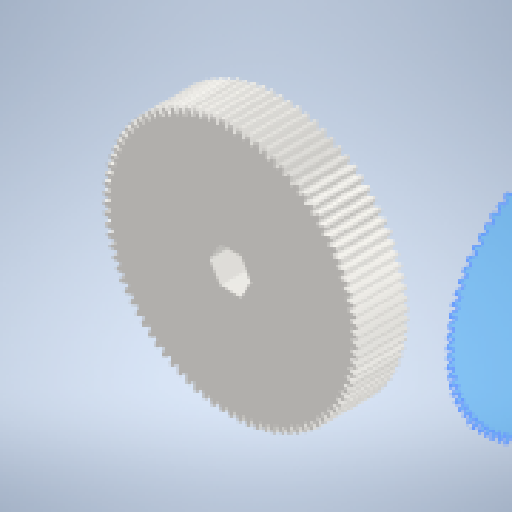
# Autodesk Inventor part: Spur Gear2
Saved by Autodesk Inventor 2024 (Build 280153020, 153B)
## iProperties
CustomPartVersion: 1
Created: 2024-04-17
Part Number: Spur Gear2
Material: Steel
Document SubType Name: Modeling
Designer: lvrectanus0
Categories: <?xml version="1.0" encoding="UTF-16"?> <MemberInstance><Categories><FamilyTemplate><FamilyTemplateParameter ValueType="xs:double" Id="1" ObjectReferenceKey="da_z" ObjectType="kUserParameterObject"/><FamilyTemplateParameter ValueType="xs:double" Id="2" ObjectReferenceKey="da_b" ObjectType="kUserParameterObject"/><FamilyTemplateParameter ValueType="xs:double" Id="3" ObjectReferenceKey="da_beta" ObjectType="kUserParameterObject"/><FamilyTemplateParameter ValueType="xs:double" Id="4" ObjectReferenceKey="da_da" ObjectType="kUserParameterObject"/><FamilyTemplateParameter ValueType="xs:double" Id="5" ObjectReferenceKey="da_aw" ObjectType="kUserParameterObject"/><FamilyTemplateParameter ValueType="xs:string" Id="6" ObjectReferenceKey="EAIAABAAAAC/AAAAAAAAAIAAAAAAAAAA" ObjectType="83910656" SubObjectId="SurfaceGeometry"/></FamilyTemplate><ParamToTemplateMap><ParamToTemplate CategoryParameter="//CategoryParameter[@InternalName='046C89C9-8512-4d59-83FE-43B91F4F132A']" TemplateParameter="1"/><ParamToTemplate CategoryParameter="//CategoryParameter[@InternalName='2552DF32-E462-4b46-AEBF-C6C7768E72AC']" TemplateParameter="2"/><ParamToTemplate CategoryParameter="//CategoryParameter[@InternalName='C9EE641D-15FC-4fae-A226-E94C4372FDD7']" TemplateParameter="3"/><ParamToTemplate><ParamToTemplate CategoryParameter="//CategoryParameter[@InternalName='00B6519A-459B-49c7-AD84-2E56D39A5744']" ConstantValue="0.000000"/></ParamToTemplate><ParamToTemplate><ParamToTemplate CategoryParameter="//CategoryParameter[@InternalName='04B31F0E-C7A6-4894-AA32-9629BEFACF47']" ConstantValue="1.000000"/></ParamToTemplate><ParamToTemplate><ParamToTemplate CategoryParameter="//CategoryParameter[@InternalName='43CBEC2E-7847-49e7-A936-2F7889FCB2D9']" ConstantValue="0.250000"/></ParamToTemplate><ParamToTemplate><ParamToTemplate CategoryParameter="//CategoryParameter[@InternalName='B1EFC894-105D-4ebd-86BF-FA20ED196853']" ConstantValue="0.350000"/></ParamToTemplate><ParamToTemplate><ParamToTemplate CategoryParameter="//CategoryParameter[@InternalName='51175063-3D10-4879-93E8-6246FE8B403D']" ConstantValue="2061532430.657340"/></ParamToTemplate><ParamToTemplate><ParamToTemplate CategoryParameter="//CategoryParameter[@InternalName='A3A52E27-4454-46a9-B0BD-C932399B70AF']" ConstantValue="0.300000"/></ParamToTemplate><ParamToTemplate><ParamToTemplate CategoryParameter="//CategoryParameter[@InternalName='91B76062-C214-41d9-B1B9-14D2AB99603D']" ConstantValue="0.079375"/></ParamToTemplate><ParamToTemplate><ParamToTemplate CategoryParameter="//CategoryParameter[@InternalName='374E806E-8B8A-4dda-A9AA-1039D6500AD2']" ConstantValue="12.598425"/></ParamToTemplate><ParamToTemplate><ParamToTemplate CategoryParameter="//CategoryParameter[@InternalName='2D373A89-B862-43d6-8D0B-0CBF12AB9F6C']" ConstantValue="0.349066"/></ParamToTemplate><ParamToTemplate CategoryParameter="//CategoryParameter[@InternalName='37777632-D6A2-4fac-9D53-DB8ACD95C989']" TemplateParameter="4"/><ParamToTemplate CategoryParameter="//CategoryParameter[@InternalName='FD1017F1-B727-4f7e-9707-0F86F1FF9423']" TemplateParameter="5"/><ParamToTemplate><ParamToTemplate CategoryParameter="//CategoryParameter[@InternalName='9E1B4470-B2D3-4ff1-B813-535BB4CDF51A']" ConstantValue="3523220.976809"/></ParamToTemplate><ParamToTemplate><ParamToTemplate CategoryParameter="//CategoryParameter[@InternalName='F8452263-BFF6-458c-9FB1-07C4B99E95CD']" ConstantValue="11397033.805607"/></ParamToTemplate><ParamToTemplate><ParamToTemplate CategoryParameter="//CategoryParameter[@InternalName='3E3BB259-FD49-497f-8171-6EBC954A3479']" ConstantValue="2.000000"/></ParamToTemplate><ParamToTemplate CategoryParameter="//CategoryParameter[@InternalName='27C3BAF2-7550-4e4b-AE2C-0DB134B7D9B7']" TemplateParameter="6"/></ParamToTemplateMap><Category DisplayName="Gear" InternalName="DC85795E-93AB-48d5-8EEE-5A27447B64BD" Mnemonic="Gear"><CategoryParameter DisplayName="z" InternalName="046C89C9-8512-4d59-83FE-43B91F4F132A" Mnemonic="z"/><CategoryParameter DisplayName="b" InternalName="2552DF32-E462-4b46-AEBF-C6C7768E72AC" Mnemonic="b"/><CategoryParameter DisplayName="||b|" InternalName="C9EE641D-15FC-4fae-A226-E94C4372FDD7" Mnemonic="beta"/><CategoryParameter DisplayName="x" InternalName="00B6519A-459B-49c7-AD84-2E56D39A5744" Mnemonic="x"/><CategoryParameter DisplayName="a*" InternalName="04B31F0E-C7A6-4894-AA32-9629BEFACF47" Mnemonic="a"/><CategoryParameter DisplayName="c*" InternalName="43CBEC2E-7847-49e7-A936-2F7889FCB2D9" Mnemonic="c"/><CategoryParameter DisplayName="r|.f|*" InternalName="B1EFC894-105D-4ebd-86BF-FA20ED196853" Mnemonic="rf"/><CategoryParameter DisplayName="E" InternalName="51175063-3D10-4879-93E8-6246FE8B403D" Mnemonic="E"/><CategoryParameter DisplayName="||m|" InternalName="A3A52E27-4454-46a9-B0BD-C932399B70AF" Mnemonic="mi"/><Category DisplayName="SpurGear" InternalName="26C5A22E-A91E-4dfd-A3B3-23CCAFAE1764" Mnemonic="SpurGear"><CategoryParameter DisplayName="m" InternalName="91B76062-C214-41d9-B1B9-14D2AB99603D" Mnemonic="m"/><CategoryParameter DisplayName="P" InternalName="374E806E-8B8A-4dda-A9AA-1039D6500AD2" Mnemonic="PP"/><CategoryParameter DisplayName="||a|" InternalName="2D373A89-B862-43d6-8D0B-0CBF12AB9F6C" Mnemonic="alpha"/><CategoryParameter DisplayName="d|.a|" InternalName="37777632-D6A2-4fac-9D53-DB8ACD95C989" Mnemonic="da"/><CategoryParameter DisplayName="a|.w|" InternalName="FD1017F1-B727-4f7e-9707-0F86F1FF9423" Mnemonic="aw"/><CategoryParameter DisplayName="||s||.Flim|" InternalName="9E1B4470-B2D3-4ff1-B813-535BB4CDF51A" Mnemonic="sFlim"/><CategoryParameter DisplayName="||s||.Hlim|" InternalName="F8452263-BFF6-458c-9FB1-07C4B99E95CD" Mnemonic="sHlim"/><CategoryParameter DisplayName="type" InternalName="3E3BB259-FD49-497f-8171-6EBC954A3479" Mnemonic="type"/><CategoryParameter DisplayName="PitchDiameter" InternalName="27C3BAF2-7550-4e4b-AE2C-0DB134B7D9B7" Mnemonic="IDS_PITCHDIAM"/></Category></Category></Categories></MemberInstance>
Density: 7.85 g/cm^3
Appearance: Steel
Mass: 494.875 g
Surface Area: 151.69 cm^2
Volume: 63.0413 cm^3
Author: lvrectanus0
Autodesk Inventor part; units mm, degrees
sketch "Sketch1" plane through (0, 0, 0) normal (0, 0, 1) x (1, 0, 0)
  circle A0 centre (0, 0) radius 37.719
  dimension "d0" = 75.438
  constraints: 1 centre point
  measures "d0" diameter of A0
extrude "Extrusion1" add sketch "Sketch1" along normal blind 15
sketch "Sketch2" plane through (0, 0, 0) normal (0, 0, -1) x (-1, 0, 0)
  circle A0 centre (0, 0) radius 37.719 projected
  circle A1 centre (0, 0) radius 36.5125
  dimension "d3" = 73.025
  constraints: 1 centre point, 1 coincident
  measures "d3" diameter of A1
surface extrude "Pitch Diameter" sketch "Sketch2" against normal through all shown no curves A1
ref_plane "Work Plane1" through (0, 0, 0) normal (1, 0, 0) x (0, 1, 0)
ref_plane "Work Plane2" through (0, 0, 0) normal (0.9993908, 0.0348995, 0) x (0, 0, 1)
ref_plane "Work Plane3" through (0, 0, 7.5) normal (0, 0, -1) x (-1, 0, 0)
spur gear teeth "Spur Gear" teeth 90 pitch diameter 73.025 tip diameter 75.438 root diameter 72.39 face width 76.2 start plane through (0, 0, 0) normal (0, 0, -1) x (-1, 0, 0)
sketch "Sketch3" plane through (0, 0, 15) normal (0, 0, 1) x (1, 0, 0)
  line L0 (-3.0383, 5.2625) -> (3.0383, 5.2625)
  line L1 (3.0383, 5.2625) -> (6.0766, 0)
  line L2 (6.0766, 0) -> (3.0383, -5.2625)
  line L3 (3.0383, -5.2625) -> (-3.0383, -5.2625)
  line L4 (-3.0383, -5.2625) -> (-6.0766, 0)
  line L5 (-6.0766, 0) -> (-3.0383, 5.2625)
  line L6 (-3.0383, 5.2625) -> (3.0383, -5.2625)
  line L7 (-6.0766, 0) -> (6.0766, 0)
  line L8 (3.0383, 5.2625) -> (-3.0383, -5.2625)
  arc A0 (-31.0852, -21.3643) -> (-29.4669, -21.0185) centre (-32.0591, -12.8456) ccw projected
  arc A1 (-29.4669, -21.0185) -> (-29.0956, -21.5296) centre (0, 0) ccw projected
  arc A2 (-29.0956, -21.5296) -> (-29.9245, -22.9619) centre (-22.1237, -26.5205) ccw projected
  arc A3 (-29.9245, -22.9619) -> (-29.5192, -23.4806) centre (0, 0) ccw projected
  arc A4 (-29.5192, -23.4806) -> (-27.929, -23.0229) centre (-31.0849, -15.0506) ccw projected
  arc A5 (-27.929, -23.0229) -> (-27.5229, -23.5068) centre (0, 0) ccw projected
  arc A6 (-27.5229, -23.5068) -> (-28.2499, -24.9934) centre (-20.2198, -27.9991) ccw projected
  arc A7 (-28.2499, -24.9934) -> (-27.8094, -25.4826) centre (0, 0) ccw projected
  arc A8 (-27.8094, -25.4826) -> (-26.2549, -24.915) centre (-29.9593, -17.1823) ccw projected
  arc A9 (-26.2549, -24.915) -> (-25.8161, -25.3694) centre (0, 0) ccw projected
  arc A10 (-25.8161, -25.3694) -> (-26.4376, -26.9031) centre (-18.2174, -29.3414) ccw projected
  arc A11 (-26.4376, -26.9031) -> (-25.964, -27.3604) centre (0, 0) ccw projected
  arc A12 (-25.964, -27.3604) -> (-24.453, -26.6858) centre (-28.6877, -19.2303) ccw projected
  arc A13 (-24.453, -26.6858) -> (-23.9835, -27.1085) centre (0, 0) ccw projected
  arc A14 (-23.9835, -27.1085) -> (-24.4965, -28.6818) centre (-16.1263, -30.5407) ccw projected
  arc A15 (-24.4965, -28.6818) -> (-23.9922, -29.1049) centre (0, 0) ccw projected
  arc A16 (-23.9922, -29.1049) -> (-22.5319, -28.3265) centre (-27.2764, -21.1846) ccw projected
  arc A17 (-22.5319, -28.3265) -> (-22.0341, -28.7154) centre (0, 0) ccw projected
  arc A18 (-22.0341, -28.7154) -> (-22.4361, -30.3207) centre (-13.9566, -31.5912) ccw projected
  arc A19 (-22.4361, -30.3207) -> (-21.9035, -30.7076) centre (0, 0) ccw projected
  arc A20 (-21.9035, -30.7076) -> (-20.5011, -29.8292) centre (-25.7322, -23.0357) ccw projected
  arc A21 (-20.5011, -29.8292) -> (-19.9774, -30.1825) centre (0, 0) ccw projected
  arc A22 (-19.9774, -30.1825) -> (-20.2664, -31.8119) centre (-11.7189, -32.4878) ccw projected
  arc A23 (-20.2664, -31.8119) -> (-19.7081, -32.1607) centre (0, 0) ccw projected
  arc A24 (-19.7081, -32.1607) -> (-18.3704, -31.1867) centre (-24.0626, -24.7746) ccw projected
  arc A25 (-18.3704, -31.1867) -> (-17.8233, -31.5025) centre (0, 0) ccw projected
  arc A26 (-17.8233, -31.5025) -> (-17.998, -33.1481) centre (-9.4241, -33.2262) ccw projected
  arc A27 (-17.998, -33.1481) -> (-17.4167, -33.4572) centre (0, 0) ccw projected
  arc A28 (-17.4167, -33.4572) -> (-16.1501, -32.3921) centre (-22.2758, -26.3928) ccw projected
  arc A29 (-16.1501, -32.3921) -> (-15.5823, -32.6691) centre (0, 0) ccw projected
  arc A30 (-15.5823, -32.6691) -> (-15.6418, -34.3228) centre (-7.0834, -33.8026) ccw projected
  arc A31 (-15.6418, -34.3228) -> (-15.0404, -34.5906) centre (0, 0) ccw projected
  arc A32 (-15.0404, -34.5906) -> (-13.8512, -33.4398) centre (-20.3805, -27.8824) ccw projected
  arc A33 (-13.8512, -33.4398) -> (-13.2655, -33.6765) centre (0, 0) ccw projected
  arc A34 (-13.2655, -33.6765) -> (-13.2095, -35.3303) centre (-4.7082, -34.2144) ccw projected
  arc A35 (-13.2095, -35.3303) -> (-12.5909, -35.5555) centre (0, 0) ccw projected
  arc A36 (-12.5909, -35.5555) -> (-11.4848, -34.3246) centre (-18.3859, -29.2361) ccw projected
  arc A37 (-11.4848, -34.3246) -> (-10.884, -34.5198) centre (0, 0) ccw projected
  arc A38 (-10.884, -34.5198) -> (-10.7128, -36.1657) centre (-2.3101, -34.4595) ccw projected
  arc A39 (-10.7128, -36.1657) -> (-10.08, -36.3472) centre (0, 0) ccw projected
  arc A40 (-10.08, -36.3472) -> (-9.0625, -35.0421) centre (-16.3017, -30.4475) ccw projected
  arc A41 (-9.0625, -35.0421) -> (-8.4496, -35.1949) centre (0, 0) ccw projected
  arc A42 (-8.4496, -35.1949) -> (-8.1639, -36.8249) centre (0.0993, -34.5367) ccw projected
  arc A43 (-8.1639, -36.8249) -> (-7.52, -36.9618) centre (0, 0) ccw projected
  arc A44 (-7.52, -36.9618) -> (-6.596, -35.5889) centre (-14.1381, -31.5104) ccw projected
  arc A45 (-6.596, -35.5889) -> (-5.9739, -35.6986) centre (0, 0) ccw projected
  arc A46 (-5.9739, -35.6986) -> (-5.5752, -37.3047) centre (2.5082, -34.4456) ccw projected
  arc A47 (-5.5752, -37.3047) -> (-4.9233, -37.3963) centre (0, 0) ccw projected
  arc A48 (-4.9233, -37.3963) -> (-4.0974, -35.9623) centre (-11.9056, -32.4199) ccw projected
  arc A49 (-4.0974, -35.9623) -> (-3.4691, -36.0284) centre (0, 0) ccw projected
  arc A50 (-3.4691, -36.0284) -> (-2.9594, -37.6027) centre (4.9049, -34.1868) ccw projected
  arc A51 (-2.9594, -37.6027) -> (-2.3027, -37.6486) centre (0, 0) ccw projected
  arc A52 (-2.3027, -37.6486) -> (-1.5788, -36.1606) centre (-9.6151, -33.1714) ccw projected
  arc A53 (-1.5788, -36.1606) -> (-0.9475, -36.1826) centre (0, 0) ccw projected
  arc A54 (-0.9475, -36.1826) -> (-0.3292, -37.7176) centre (7.2777, -33.7613) ccw projected
  arc A55 (-0.3292, -37.7176) -> (0.3292, -37.7176) centre (0, 0) ccw projected
  arc A56 (0.3292, -37.7176) -> (0.9475, -36.1826) centre (-7.2777, -33.7613) ccw projected
  arc A57 (0.9475, -36.1826) -> (1.5788, -36.1606) centre (0, 0) ccw projected
  arc A58 (1.5788, -36.1606) -> (2.3027, -37.6486) centre (9.6151, -33.1714) ccw projected
  arc A59 (2.3027, -37.6486) -> (2.9594, -37.6027) centre (0, 0) ccw projected
  arc A60 (2.9594, -37.6027) -> (3.4691, -36.0284) centre (-4.9049, -34.1868) ccw projected
  arc A61 (3.4691, -36.0284) -> (4.0974, -35.9623) centre (0, 0) ccw projected
  arc A62 (4.0974, -35.9623) -> (4.9233, -37.3963) centre (11.9056, -32.4199) ccw projected
  arc A63 (4.9233, -37.3963) -> (5.5752, -37.3047) centre (0, 0) ccw projected
  arc A64 (5.5752, -37.3047) -> (5.9739, -35.6986) centre (-2.5082, -34.4456) ccw projected
  arc A65 (5.9739, -35.6986) -> (6.596, -35.5889) centre (0, 0) ccw projected
  arc A66 (6.596, -35.5889) -> (7.52, -36.9618) centre (14.1381, -31.5104) ccw projected
  arc A67 (7.52, -36.9618) -> (8.1639, -36.8249) centre (0, 0) ccw projected
  arc A68 (8.1639, -36.8249) -> (8.4496, -35.1949) centre (-0.0993, -34.5367) ccw projected
  arc A69 (8.4496, -35.1949) -> (9.0625, -35.0421) centre (0, 0) ccw projected
  arc A70 (9.0625, -35.0421) -> (10.08, -36.3472) centre (16.3017, -30.4475) ccw projected
  arc A71 (10.08, -36.3472) -> (10.7128, -36.1657) centre (0, 0) ccw projected
  arc A72 (10.7128, -36.1657) -> (10.884, -34.5198) centre (2.3101, -34.4595) ccw projected
  arc A73 (10.884, -34.5198) -> (11.4848, -34.3246) centre (0, 0) ccw projected
  arc A74 (11.4848, -34.3246) -> (12.5909, -35.5555) centre (18.3859, -29.2361) ccw projected
  arc A75 (12.5909, -35.5555) -> (13.2095, -35.3303) centre (0, 0) ccw projected
  arc A76 (13.2095, -35.3303) -> (13.2655, -33.6765) centre (4.7082, -34.2144) ccw projected
  arc A77 (13.2655, -33.6765) -> (13.8512, -33.4398) centre (0, 0) ccw projected
  arc A78 (13.8512, -33.4398) -> (15.0404, -34.5906) centre (20.3805, -27.8824) ccw projected
  arc A79 (15.0404, -34.5906) -> (15.6418, -34.3228) centre (0, 0) ccw projected
  arc A80 (15.6418, -34.3228) -> (15.5823, -32.6691) centre (7.0834, -33.8026) ccw projected
  arc A81 (15.5823, -32.6691) -> (16.1501, -32.3921) centre (0, 0) ccw projected
  arc A82 (16.1501, -32.3921) -> (17.4167, -33.4572) centre (22.2758, -26.3928) ccw projected
  arc A83 (17.4167, -33.4572) -> (17.998, -33.1481) centre (0, 0) ccw projected
  arc A84 (17.998, -33.1481) -> (17.8233, -31.5025) centre (9.4241, -33.2262) ccw projected
  arc A85 (17.8233, -31.5025) -> (18.3704, -31.1867) centre (0, 0) ccw projected
  arc A86 (18.3704, -31.1867) -> (19.7081, -32.1607) centre (24.0626, -24.7746) ccw projected
  arc A87 (19.7081, -32.1607) -> (20.2664, -31.8119) centre (0, 0) ccw projected
  arc A88 (20.2664, -31.8119) -> (19.9774, -30.1825) centre (11.7189, -32.4878) ccw projected
  arc A89 (19.9774, -30.1825) -> (20.5011, -29.8292) centre (0, 0) ccw projected
  arc A90 (20.5011, -29.8292) -> (21.9035, -30.7076) centre (25.7322, -23.0357) ccw projected
  arc A91 (21.9035, -30.7076) -> (22.4361, -30.3207) centre (0, 0) ccw projected
  arc A92 (22.4361, -30.3207) -> (22.0341, -28.7154) centre (13.9566, -31.5912) ccw projected
  arc A93 (22.0341, -28.7154) -> (22.5319, -28.3265) centre (0, 0) ccw projected
  arc A94 (22.5319, -28.3265) -> (23.9922, -29.1049) centre (27.2764, -21.1846) ccw projected
  arc A95 (23.9922, -29.1049) -> (24.4965, -28.6818) centre (0, 0) ccw projected
  arc A96 (24.4965, -28.6818) -> (23.9835, -27.1085) centre (16.1263, -30.5407) ccw projected
  arc A97 (23.9835, -27.1085) -> (24.453, -26.6858) centre (0, 0) ccw projected
  arc A98 (24.453, -26.6858) -> (25.964, -27.3604) centre (28.6877, -19.2303) ccw projected
  arc A99 (25.964, -27.3604) -> (26.4376, -26.9031) centre (0, 0) ccw projected
  arc A100 (26.4376, -26.9031) -> (25.8161, -25.3694) centre (18.2174, -29.3414) ccw projected
  arc A101 (25.8161, -25.3694) -> (26.2549, -24.915) centre (0, 0) ccw projected
  arc A102 (26.2549, -24.915) -> (27.8094, -25.4826) centre (29.9593, -17.1823) ccw projected
  arc A103 (27.8094, -25.4826) -> (28.2499, -24.9934) centre (0, 0) ccw projected
  arc A104 (28.2499, -24.9934) -> (27.5229, -23.5068) centre (20.2198, -27.9991) ccw projected
  arc A105 (27.5229, -23.5068) -> (27.929, -23.0229) centre (0, 0) ccw projected
  arc A106 (27.929, -23.0229) -> (29.5192, -23.4806) centre (31.0849, -15.0506) ccw projected
  arc A107 (29.5192, -23.4806) -> (29.9245, -22.9619) centre (0, 0) ccw projected
  arc A108 (29.9245, -22.9619) -> (29.0956, -21.5296) centre (22.1237, -26.5205) ccw projected
  arc A109 (29.0956, -21.5296) -> (29.4669, -21.0185) centre (0, 0) ccw projected
  arc A110 (29.4669, -21.0185) -> (31.0852, -21.3643) centre (32.0591, -12.8456) ccw projected
  arc A111 (31.0852, -21.3643) -> (31.4533, -20.8185) centre (0, 0) ccw projected
  arc A112 (31.4533, -20.8185) -> (30.5266, -19.4476) centre (23.9198, -24.9126) ccw projected
  arc A113 (30.5266, -19.4476) -> (30.8613, -18.9118) centre (0, 0) ccw projected
  arc A114 (30.8613, -18.9118) -> (32.4998, -19.1438) centre (32.877, -10.578) ccw projected
  arc A115 (32.4998, -19.1438) -> (32.8289, -18.5737) centre (0, 0) ccw projected
  arc A116 (32.8289, -18.5737) -> (31.8088, -17.2708) centre (25.5993, -23.1834) ccw projected
  arc A117 (31.8088, -17.2708) -> (32.1054, -16.713) centre (0, 0) ccw projected
  arc A118 (32.1054, -16.713) -> (33.756, -16.8301) centre (33.5348, -8.2588) ccw projected
  arc A119 (33.756, -16.8301) -> (34.0446, -16.2384) centre (0, 0) ccw projected
  arc A120 (34.0446, -16.2384) -> (32.936, -15.0098) centre (27.1541, -21.3412) ccw projected
  arc A121 (32.936, -15.0098) -> (33.193, -14.4327) centre (0, 0) ccw projected
  arc A122 (33.193, -14.4327) -> (34.8478, -14.4344) centre (34.0292, -5.8994) ccw projected
  arc A123 (34.8478, -14.4344) -> (35.0944, -13.8241) centre (0, 0) ccw projected
  arc A124 (35.0944, -13.8241) -> (33.9028, -12.6758) centre (28.5767, -19.395) ccw projected
  arc A125 (33.9028, -12.6758) -> (34.1189, -12.0821) centre (0, 0) ccw projected
  arc A126 (34.1189, -12.0821) -> (35.7698, -11.9684) centre (34.3579, -3.5113) ccw projected
  arc A127 (35.7698, -11.9684) -> (35.9732, -11.3423) centre (0, 0) ccw projected
  arc A128 (35.9732, -11.3423) -> (34.7045, -10.2799) centre (29.86, -17.3543) ccw projected
  arc A129 (34.7045, -10.2799) -> (34.8786, -9.6727) centre (0, 0) ccw projected
  arc A130 (34.8786, -9.6727) -> (36.5176, -9.4441) centre (34.5191, -1.1061) ccw projected
  arc A131 (36.5176, -9.4441) -> (36.6768, -8.8053) centre (0, 0) ccw projected
  arc A132 (36.6768, -8.8053) -> (35.337, -7.834) centre (30.9978, -15.2291) ccw projected
  arc A133 (35.337, -7.834) -> (35.4684, -7.2161) centre (0, 0) ccw projected
  arc A134 (35.4684, -7.2161) -> (37.0874, -6.8737) centre (34.5122, 1.3046) ccw projected
  arc A135 (37.0874, -6.8737) -> (37.2017, -6.2254) centre (0, 0) ccw projected
  arc A136 (37.2017, -6.2254) -> (35.7974, -5.35) centre (31.9847, -13.0298) ccw projected
  arc A137 (35.7974, -5.35) -> (35.8853, -4.7244) centre (0, 0) ccw projected
  arc A138 (35.8853, -4.7244) -> (37.4765, -4.2699) centre (34.3371, 3.7088) ccw projected
  arc A139 (37.4765, -4.2699) -> (37.5453, -3.6152) centre (0, 0) ccw projected
  arc A140 (37.5453, -3.6152) -> (36.0834, -2.8398) centre (32.8156, -10.7669) ccw projected
  arc A141 (36.0834, -2.8398) -> (36.1275, -2.2097) centre (0, 0) ccw projected
  arc A142 (36.1275, -2.2097) -> (37.6831, -1.6453) centre (33.9947, 6.095) ccw projected
  arc A143 (37.6831, -1.6453) -> (37.7061, -0.9874) centre (0, 0) ccw projected
  arc A144 (37.7061, -0.9874) -> (36.1936, -0.3159) centre (33.4868, -8.4515) ccw projected
  arc A145 (36.1936, -0.3159) -> (36.1936, 0.3159) centre (0, 0) ccw projected
  arc A146 (36.1936, 0.3159) -> (37.7061, 0.9874) centre (33.4868, 8.4515) ccw projected
  arc A147 (37.7061, 0.9874) -> (37.6831, 1.6453) centre (0, 0) ccw projected
  arc A148 (37.6831, 1.6453) -> (36.1275, 2.2097) centre (33.9947, -6.095) ccw projected
  arc A149 (36.1275, 2.2097) -> (36.0834, 2.8398) centre (0, 0) ccw projected
  arc A150 (36.0834, 2.8398) -> (37.5453, 3.6152) centre (32.8156, 10.7669) ccw projected
  arc A151 (37.5453, 3.6152) -> (37.4765, 4.2699) centre (0, 0) ccw projected
  arc A152 (37.4765, 4.2699) -> (35.8853, 4.7244) centre (34.3371, -3.7088) ccw projected
  arc A153 (35.8853, 4.7244) -> (35.7974, 5.35) centre (0, 0) ccw projected
  arc A154 (35.7974, 5.35) -> (37.2017, 6.2254) centre (31.9847, 13.0298) ccw projected
  arc A155 (37.2017, 6.2254) -> (37.0874, 6.8737) centre (0, 0) ccw projected
  arc A156 (37.0874, 6.8737) -> (35.4684, 7.2161) centre (34.5122, -1.3046) ccw projected
  arc A157 (35.4684, 7.2161) -> (35.337, 7.834) centre (0, 0) ccw projected
  arc A158 (35.337, 7.834) -> (36.6768, 8.8053) centre (30.9978, 15.2291) ccw projected
  arc A159 (36.6768, 8.8053) -> (36.5176, 9.4441) centre (0, 0) ccw projected
  arc A160 (36.5176, 9.4441) -> (34.8786, 9.6727) centre (34.5191, 1.1061) ccw projected
  arc A161 (34.8786, 9.6727) -> (34.7045, 10.2799) centre (0, 0) ccw projected
  arc A162 (34.7045, 10.2799) -> (35.9732, 11.3423) centre (29.86, 17.3543) ccw projected
  arc A163 (35.9732, 11.3423) -> (35.7698, 11.9684) centre (0, 0) ccw projected
  arc A164 (35.7698, 11.9684) -> (34.1189, 12.0821) centre (34.3579, 3.5113) ccw projected
  arc A165 (34.1189, 12.0821) -> (33.9028, 12.6758) centre (0, 0) ccw projected
  arc A166 (33.9028, 12.6758) -> (35.0944, 13.8241) centre (28.5767, 19.395) ccw projected
  arc A167 (35.0944, 13.8241) -> (34.8478, 14.4344) centre (0, 0) ccw projected
  arc A168 (34.8478, 14.4344) -> (33.193, 14.4327) centre (34.0292, 5.8994) ccw projected
  arc A169 (33.193, 14.4327) -> (32.936, 15.0098) centre (0, 0) ccw projected
  arc A170 (32.936, 15.0098) -> (34.0446, 16.2384) centre (27.1541, 21.3412) ccw projected
  arc A171 (34.0446, 16.2384) -> (33.756, 16.8301) centre (0, 0) ccw projected
  arc A172 (33.756, 16.8301) -> (32.1054, 16.713) centre (33.5348, 8.2588) ccw projected
  arc A173 (32.1054, 16.713) -> (31.8088, 17.2708) centre (0, 0) ccw projected
  arc A174 (31.8088, 17.2708) -> (32.8289, 18.5737) centre (25.5993, 23.1834) ccw projected
  arc A175 (32.8289, 18.5737) -> (32.4998, 19.1438) centre (0, 0) ccw projected
  arc A176 (32.4998, 19.1438) -> (30.8613, 18.9118) centre (32.877, 10.578) ccw projected
  arc A177 (30.8613, 18.9118) -> (30.5266, 19.4476) centre (0, 0) ccw projected
  arc A178 (30.5266, 19.4476) -> (31.4533, 20.8185) centre (23.9198, 24.9126) ccw projected
  arc A179 (31.4533, 20.8185) -> (31.0852, 21.3643) centre (0, 0) ccw projected
  arc A180 (31.0852, 21.3643) -> (29.4669, 21.0185) centre (32.0591, 12.8456) ccw projected
  arc A181 (29.4669, 21.0185) -> (29.0956, 21.5296) centre (0, 0) ccw projected
  arc A182 (29.0956, 21.5296) -> (29.9245, 22.9619) centre (22.1237, 26.5205) ccw projected
  arc A183 (29.9245, 22.9619) -> (29.5192, 23.4806) centre (0, 0) ccw projected
  arc A184 (29.5192, 23.4806) -> (27.929, 23.0229) centre (31.0849, 15.0506) ccw projected
  arc A185 (27.929, 23.0229) -> (27.5229, 23.5068) centre (0, 0) ccw projected
  arc A186 (27.5229, 23.5068) -> (28.2499, 24.9934) centre (20.2198, 27.9991) ccw projected
  arc A187 (28.2499, 24.9934) -> (27.8094, 25.4826) centre (0, 0) ccw projected
  arc A188 (27.8094, 25.4826) -> (26.2549, 24.915) centre (29.9593, 17.1823) ccw projected
  arc A189 (26.2549, 24.915) -> (25.8161, 25.3694) centre (0, 0) ccw projected
  arc A190 (25.8161, 25.3694) -> (26.4376, 26.9031) centre (18.2174, 29.3414) ccw projected
  arc A191 (26.4376, 26.9031) -> (25.964, 27.3604) centre (0, 0) ccw projected
  arc A192 (25.964, 27.3604) -> (24.453, 26.6858) centre (28.6877, 19.2303) ccw projected
  arc A193 (24.453, 26.6858) -> (23.9835, 27.1085) centre (0, 0) ccw projected
  arc A194 (23.9835, 27.1085) -> (24.4965, 28.6818) centre (16.1263, 30.5407) ccw projected
  arc A195 (24.4965, 28.6818) -> (23.9922, 29.1049) centre (0, 0) ccw projected
  arc A196 (23.9922, 29.1049) -> (22.5319, 28.3265) centre (27.2764, 21.1846) ccw projected
  arc A197 (22.5319, 28.3265) -> (22.0341, 28.7154) centre (0, 0) ccw projected
  arc A198 (22.0341, 28.7154) -> (22.4361, 30.3207) centre (13.9566, 31.5912) ccw projected
  arc A199 (22.4361, 30.3207) -> (21.9035, 30.7076) centre (0, 0) ccw projected
  arc A200 (21.9035, 30.7076) -> (20.5011, 29.8292) centre (25.7322, 23.0357) ccw projected
  arc A201 (20.5011, 29.8292) -> (19.9774, 30.1825) centre (0, 0) ccw projected
  arc A202 (19.9774, 30.1825) -> (20.2664, 31.8119) centre (11.7189, 32.4878) ccw projected
  arc A203 (20.2664, 31.8119) -> (19.7081, 32.1607) centre (0, 0) ccw projected
  arc A204 (19.7081, 32.1607) -> (18.3704, 31.1867) centre (24.0626, 24.7746) ccw projected
  arc A205 (18.3704, 31.1867) -> (17.8233, 31.5025) centre (0, 0) ccw projected
  arc A206 (17.8233, 31.5025) -> (17.998, 33.1481) centre (9.4241, 33.2262) ccw projected
  arc A207 (17.998, 33.1481) -> (17.4167, 33.4572) centre (0, 0) ccw projected
  arc A208 (17.4167, 33.4572) -> (16.1501, 32.3921) centre (22.2758, 26.3928) ccw projected
  arc A209 (16.1501, 32.3921) -> (15.5823, 32.6691) centre (0, 0) ccw projected
  arc A210 (15.5823, 32.6691) -> (15.6418, 34.3228) centre (7.0834, 33.8026) ccw projected
  arc A211 (15.6418, 34.3228) -> (15.0404, 34.5906) centre (0, 0) ccw projected
  arc A212 (15.0404, 34.5906) -> (13.8512, 33.4398) centre (20.3805, 27.8824) ccw projected
  arc A213 (13.8512, 33.4398) -> (13.2655, 33.6765) centre (0, 0) ccw projected
  arc A214 (13.2655, 33.6765) -> (13.2095, 35.3303) centre (4.7082, 34.2144) ccw projected
  arc A215 (13.2095, 35.3303) -> (12.5909, 35.5555) centre (0, 0) ccw projected
  arc A216 (12.5909, 35.5555) -> (11.4848, 34.3246) centre (18.3859, 29.2361) ccw projected
  arc A217 (11.4848, 34.3246) -> (10.884, 34.5198) centre (0, 0) ccw projected
  arc A218 (10.884, 34.5198) -> (10.7128, 36.1657) centre (2.3101, 34.4595) ccw projected
  arc A219 (10.7128, 36.1657) -> (10.08, 36.3472) centre (0, 0) ccw projected
  arc A220 (10.08, 36.3472) -> (9.0625, 35.0421) centre (16.3017, 30.4475) ccw projected
  arc A221 (9.0625, 35.0421) -> (8.4496, 35.1949) centre (0, 0) ccw projected
  arc A222 (8.4496, 35.1949) -> (8.1639, 36.8249) centre (-0.0993, 34.5367) ccw projected
  arc A223 (8.1639, 36.8249) -> (7.52, 36.9618) centre (0, 0) ccw projected
  arc A224 (7.52, 36.9618) -> (6.596, 35.5889) centre (14.1381, 31.5104) ccw projected
  arc A225 (6.596, 35.5889) -> (5.9739, 35.6986) centre (0, 0) ccw projected
  arc A226 (5.9739, 35.6986) -> (5.5752, 37.3047) centre (-2.5082, 34.4456) ccw projected
  arc A227 (5.5752, 37.3047) -> (4.9233, 37.3963) centre (0, 0) ccw projected
  arc A228 (4.9233, 37.3963) -> (4.0974, 35.9623) centre (11.9056, 32.4199) ccw projected
  arc A229 (4.0974, 35.9623) -> (3.4691, 36.0284) centre (0, 0) ccw projected
  arc A230 (3.4691, 36.0284) -> (2.9594, 37.6027) centre (-4.9049, 34.1868) ccw projected
  arc A231 (2.9594, 37.6027) -> (2.3027, 37.6486) centre (0, 0) ccw projected
  arc A232 (2.3027, 37.6486) -> (1.5788, 36.1606) centre (9.6151, 33.1714) ccw projected
  arc A233 (1.5788, 36.1606) -> (0.9475, 36.1826) centre (0, 0) ccw projected
  arc A234 (0.9475, 36.1826) -> (0.3292, 37.7176) centre (-7.2777, 33.7613) ccw projected
  arc A235 (0.3292, 37.7176) -> (-0.3292, 37.7176) centre (0, 0) ccw projected
  arc A236 (-0.3292, 37.7176) -> (-0.9475, 36.1826) centre (7.2777, 33.7613) ccw projected
  arc A237 (-0.9475, 36.1826) -> (-1.5788, 36.1606) centre (0, 0) ccw projected
  arc A238 (-1.5788, 36.1606) -> (-2.3027, 37.6486) centre (-9.6151, 33.1714) ccw projected
  arc A239 (-31.4533, -20.8185) -> (-31.0852, -21.3643) centre (0, 0) ccw projected
  arc A240 (-2.9594, 37.6027) -> (-3.4691, 36.0284) centre (4.9049, 34.1868) ccw projected
  arc A241 (-3.4691, 36.0284) -> (-4.0974, 35.9623) centre (0, 0) ccw projected
  arc A242 (-4.0974, 35.9623) -> (-4.9233, 37.3963) centre (-11.9056, 32.4199) ccw projected
  arc A243 (-4.9233, 37.3963) -> (-5.5752, 37.3047) centre (0, 0) ccw projected
  arc A244 (-5.5752, 37.3047) -> (-5.9739, 35.6986) centre (2.5082, 34.4456) ccw projected
  arc A245 (-5.9739, 35.6986) -> (-6.596, 35.5889) centre (0, 0) ccw projected
  arc A246 (-6.596, 35.5889) -> (-7.52, 36.9618) centre (-14.1381, 31.5104) ccw projected
  arc A247 (-7.52, 36.9618) -> (-8.1639, 36.8249) centre (0, 0) ccw projected
  arc A248 (-8.1639, 36.8249) -> (-8.4496, 35.1949) centre (0.0993, 34.5367) ccw projected
  arc A249 (-8.4496, 35.1949) -> (-9.0625, 35.0421) centre (0, 0) ccw projected
  arc A250 (-9.0625, 35.0421) -> (-10.08, 36.3472) centre (-16.3017, 30.4475) ccw projected
  arc A251 (-10.08, 36.3472) -> (-10.7128, 36.1657) centre (0, 0) ccw projected
  arc A252 (-10.7128, 36.1657) -> (-10.884, 34.5198) centre (-2.3101, 34.4595) ccw projected
  arc A253 (-10.884, 34.5198) -> (-11.4848, 34.3246) centre (0, 0) ccw projected
  arc A254 (-11.4848, 34.3246) -> (-12.5909, 35.5555) centre (-18.3859, 29.2361) ccw projected
  arc A255 (-12.5909, 35.5555) -> (-13.2095, 35.3303) centre (0, 0) ccw projected
  arc A256 (-13.2095, 35.3303) -> (-13.2655, 33.6765) centre (-4.7082, 34.2144) ccw projected
  arc A257 (-13.2655, 33.6765) -> (-13.8512, 33.4398) centre (0, 0) ccw projected
  arc A258 (-13.8512, 33.4398) -> (-15.0404, 34.5906) centre (-20.3805, 27.8824) ccw projected
  arc A259 (-15.0404, 34.5906) -> (-15.6418, 34.3228) centre (0, 0) ccw projected
  arc A260 (-15.6418, 34.3228) -> (-15.5823, 32.6691) centre (-7.0834, 33.8026) ccw projected
  arc A261 (-15.5823, 32.6691) -> (-16.1501, 32.3921) centre (0, 0) ccw projected
  arc A262 (-16.1501, 32.3921) -> (-17.4167, 33.4572) centre (-22.2758, 26.3928) ccw projected
  arc A263 (-17.4167, 33.4572) -> (-17.998, 33.1481) centre (0, 0) ccw projected
  arc A264 (-17.998, 33.1481) -> (-17.8233, 31.5025) centre (-9.4241, 33.2262) ccw projected
  arc A265 (-17.8233, 31.5025) -> (-18.3704, 31.1867) centre (0, 0) ccw projected
  arc A266 (-18.3704, 31.1867) -> (-19.7081, 32.1607) centre (-24.0626, 24.7746) ccw projected
  arc A267 (-19.7081, 32.1607) -> (-20.2664, 31.8119) centre (0, 0) ccw projected
  arc A268 (-20.2664, 31.8119) -> (-19.9774, 30.1825) centre (-11.7189, 32.4878) ccw projected
  arc A269 (-19.9774, 30.1825) -> (-20.5011, 29.8292) centre (0, 0) ccw projected
  arc A270 (-20.5011, 29.8292) -> (-21.9035, 30.7076) centre (-25.7322, 23.0357) ccw projected
  arc A271 (-21.9035, 30.7076) -> (-22.4361, 30.3207) centre (0, 0) ccw projected
  arc A272 (-22.4361, 30.3207) -> (-22.0341, 28.7154) centre (-13.9566, 31.5912) ccw projected
  arc A273 (-22.0341, 28.7154) -> (-22.5319, 28.3265) centre (0, 0) ccw projected
  arc A274 (-22.5319, 28.3265) -> (-23.9922, 29.1049) centre (-27.2764, 21.1846) ccw projected
  arc A275 (-23.9922, 29.1049) -> (-24.4965, 28.6818) centre (0, 0) ccw projected
  arc A276 (-24.4965, 28.6818) -> (-23.9835, 27.1085) centre (-16.1263, 30.5407) ccw projected
  arc A277 (-23.9835, 27.1085) -> (-24.453, 26.6858) centre (0, 0) ccw projected
  arc A278 (-24.453, 26.6858) -> (-25.964, 27.3604) centre (-28.6877, 19.2303) ccw projected
  arc A279 (-25.964, 27.3604) -> (-26.4376, 26.9031) centre (0, 0) ccw projected
  arc A280 (-26.4376, 26.9031) -> (-25.8161, 25.3694) centre (-18.2174, 29.3414) ccw projected
  arc A281 (-25.8161, 25.3694) -> (-26.2549, 24.915) centre (0, 0) ccw projected
  arc A282 (-26.2549, 24.915) -> (-27.8094, 25.4826) centre (-29.9593, 17.1823) ccw projected
  arc A283 (-27.8094, 25.4826) -> (-28.2499, 24.9934) centre (0, 0) ccw projected
  arc A284 (-28.2499, 24.9934) -> (-27.5229, 23.5068) centre (-20.2198, 27.9991) ccw projected
  arc A285 (-27.5229, 23.5068) -> (-27.929, 23.0229) centre (0, 0) ccw projected
  arc A286 (-27.929, 23.0229) -> (-29.5192, 23.4806) centre (-31.0849, 15.0506) ccw projected
  arc A287 (-29.5192, 23.4806) -> (-29.9245, 22.9619) centre (0, 0) ccw projected
  arc A288 (-29.9245, 22.9619) -> (-29.0956, 21.5296) centre (-22.1237, 26.5205) ccw projected
  arc A289 (-29.0956, 21.5296) -> (-29.4669, 21.0185) centre (0, 0) ccw projected
  arc A290 (-29.4669, 21.0185) -> (-31.0852, 21.3643) centre (-32.0591, 12.8456) ccw projected
  arc A291 (-31.0852, 21.3643) -> (-31.4533, 20.8185) centre (0, 0) ccw projected
  arc A292 (-31.4533, 20.8185) -> (-30.5266, 19.4476) centre (-23.9198, 24.9126) ccw projected
  arc A293 (-30.5266, 19.4476) -> (-30.8613, 18.9118) centre (0, 0) ccw projected
  arc A294 (-30.8613, 18.9118) -> (-32.4998, 19.1438) centre (-32.877, 10.578) ccw projected
  arc A295 (-32.4998, 19.1438) -> (-32.8289, 18.5737) centre (0, 0) ccw projected
  arc A296 (-32.8289, 18.5737) -> (-31.8088, 17.2708) centre (-25.5993, 23.1834) ccw projected
  arc A297 (-31.8088, 17.2708) -> (-32.1054, 16.713) centre (0, 0) ccw projected
  arc A298 (-32.1054, 16.713) -> (-33.756, 16.8301) centre (-33.5348, 8.2588) ccw projected
  arc A299 (-33.756, 16.8301) -> (-34.0446, 16.2384) centre (0, 0) ccw projected
  arc A300 (-34.0446, 16.2384) -> (-32.936, 15.0098) centre (-27.1541, 21.3412) ccw projected
  arc A301 (-32.936, 15.0098) -> (-33.193, 14.4327) centre (0, 0) ccw projected
  arc A302 (-33.193, 14.4327) -> (-34.8478, 14.4344) centre (-34.0292, 5.8994) ccw projected
  arc A303 (-34.8478, 14.4344) -> (-35.0944, 13.8241) centre (0, 0) ccw projected
  arc A304 (-35.0944, 13.8241) -> (-33.9028, 12.6758) centre (-28.5767, 19.395) ccw projected
  arc A305 (-33.9028, 12.6758) -> (-34.1189, 12.0821) centre (0, 0) ccw projected
  arc A306 (-34.1189, 12.0821) -> (-35.7698, 11.9684) centre (-34.3579, 3.5113) ccw projected
  arc A307 (-35.7698, 11.9684) -> (-35.9732, 11.3423) centre (0, 0) ccw projected
  arc A308 (-35.9732, 11.3423) -> (-34.7045, 10.2799) centre (-29.86, 17.3543) ccw projected
  arc A309 (-34.7045, 10.2799) -> (-34.8786, 9.6727) centre (0, 0) ccw projected
  arc A310 (-34.8786, 9.6727) -> (-36.5176, 9.4441) centre (-34.5191, 1.1061) ccw projected
  arc A311 (-36.5176, 9.4441) -> (-36.6768, 8.8053) centre (0, 0) ccw projected
  arc A312 (-36.6768, 8.8053) -> (-35.337, 7.834) centre (-30.9978, 15.2291) ccw projected
  arc A313 (-35.337, 7.834) -> (-35.4684, 7.2161) centre (0, 0) ccw projected
  arc A314 (-35.4684, 7.2161) -> (-37.0874, 6.8737) centre (-34.5122, -1.3046) ccw projected
  arc A315 (-37.0874, 6.8737) -> (-37.2017, 6.2254) centre (0, 0) ccw projected
  arc A316 (-37.2017, 6.2254) -> (-35.7974, 5.35) centre (-31.9847, 13.0298) ccw projected
  arc A317 (-35.7974, 5.35) -> (-35.8853, 4.7244) centre (0, 0) ccw projected
  arc A318 (-35.8853, 4.7244) -> (-37.4765, 4.2699) centre (-34.3371, -3.7088) ccw projected
  arc A319 (-37.4765, 4.2699) -> (-37.5453, 3.6152) centre (0, 0) ccw projected
  arc A320 (-37.5453, 3.6152) -> (-36.0834, 2.8398) centre (-32.8156, 10.7669) ccw projected
  arc A321 (-36.0834, 2.8398) -> (-36.1275, 2.2097) centre (0, 0) ccw projected
  arc A322 (-36.1275, 2.2097) -> (-37.6831, 1.6453) centre (-33.9947, -6.095) ccw projected
  arc A323 (-37.6831, 1.6453) -> (-37.7061, 0.9874) centre (0, 0) ccw projected
  arc A324 (-37.7061, 0.9874) -> (-36.1936, 0.3159) centre (-33.4868, 8.4515) ccw projected
  arc A325 (-36.1936, 0.3159) -> (-36.1936, -0.3159) centre (0, 0) ccw projected
  arc A326 (-36.1936, -0.3159) -> (-37.7061, -0.9874) centre (-33.4868, -8.4515) ccw projected
  arc A327 (-37.7061, -0.9874) -> (-37.6831, -1.6453) centre (0, 0) ccw projected
  arc A328 (-37.6831, -1.6453) -> (-36.1275, -2.2097) centre (-33.9947, 6.095) ccw projected
  arc A329 (-36.1275, -2.2097) -> (-36.0834, -2.8398) centre (0, 0) ccw projected
  arc A330 (-36.0834, -2.8398) -> (-37.5453, -3.6152) centre (-32.8156, -10.7669) ccw projected
  arc A331 (-37.5453, -3.6152) -> (-37.4765, -4.2699) centre (0, 0) ccw projected
  arc A332 (-37.4765, -4.2699) -> (-35.8853, -4.7244) centre (-34.3371, 3.7088) ccw projected
  arc A333 (-35.8853, -4.7244) -> (-35.7974, -5.35) centre (0, 0) ccw projected
  arc A334 (-35.7974, -5.35) -> (-37.2017, -6.2254) centre (-31.9847, -13.0298) ccw projected
  arc A335 (-37.2017, -6.2254) -> (-37.0874, -6.8737) centre (0, 0) ccw projected
  arc A336 (-37.0874, -6.8737) -> (-35.4684, -7.2161) centre (-34.5122, 1.3046) ccw projected
  arc A337 (-35.4684, -7.2161) -> (-35.337, -7.834) centre (0, 0) ccw projected
  arc A338 (-35.337, -7.834) -> (-36.6768, -8.8053) centre (-30.9978, -15.2291) ccw projected
  arc A339 (-36.6768, -8.8053) -> (-36.5176, -9.4441) centre (0, 0) ccw projected
  arc A340 (-36.5176, -9.4441) -> (-34.8786, -9.6727) centre (-34.5191, -1.1061) ccw projected
  arc A341 (-34.8786, -9.6727) -> (-34.7045, -10.2799) centre (0, 0) ccw projected
  arc A342 (-34.7045, -10.2799) -> (-35.9732, -11.3423) centre (-29.86, -17.3543) ccw projected
  arc A343 (-35.9732, -11.3423) -> (-35.7698, -11.9684) centre (0, 0) ccw projected
  arc A344 (-35.7698, -11.9684) -> (-34.1189, -12.0821) centre (-34.3579, -3.5113) ccw projected
  arc A345 (-34.1189, -12.0821) -> (-33.9028, -12.6758) centre (0, 0) ccw projected
  arc A346 (-33.9028, -12.6758) -> (-35.0944, -13.8241) centre (-28.5767, -19.395) ccw projected
  arc A347 (-35.0944, -13.8241) -> (-34.8478, -14.4344) centre (0, 0) ccw projected
  arc A348 (-34.8478, -14.4344) -> (-33.193, -14.4327) centre (-34.0292, -5.8994) ccw projected
  arc A349 (-33.193, -14.4327) -> (-32.936, -15.0098) centre (0, 0) ccw projected
  arc A350 (-32.936, -15.0098) -> (-34.0446, -16.2384) centre (-27.1541, -21.3412) ccw projected
  arc A351 (-34.0446, -16.2384) -> (-33.756, -16.8301) centre (0, 0) ccw projected
  arc A352 (-33.756, -16.8301) -> (-32.1054, -16.713) centre (-33.5348, -8.2588) ccw projected
  arc A353 (-32.1054, -16.713) -> (-31.8088, -17.2708) centre (0, 0) ccw projected
  arc A354 (-31.8088, -17.2708) -> (-32.8289, -18.5737) centre (-25.5993, -23.1834) ccw projected
  arc A355 (-32.8289, -18.5737) -> (-32.4998, -19.1438) centre (0, 0) ccw projected
  arc A356 (-32.4998, -19.1438) -> (-30.8613, -18.9118) centre (-32.877, -10.578) ccw projected
  arc A357 (-30.8613, -18.9118) -> (-30.5266, -19.4476) centre (0, 0) ccw projected
  arc A358 (-30.5266, -19.4476) -> (-31.4533, -20.8185) centre (-23.9198, -24.9126) ccw projected
  arc A359 (-2.3027, 37.6486) -> (-2.9594, 37.6027) centre (0, 0) ccw projected
  dimension "d21" = 10.525
  dimension "d22" = 10.525
  dimension "d23" = 10.525
  constraints: 18 end point, 3 equal length, 1 coincident, 1 horizontal, 1 midpoint, 1 parallel
  measures "d21" distance between parallel lines of L3 L0
  measures "d22" distance between parallel lines of L4 L1
  measures "d23" distance between parallel lines of L2 L5
extrude "Extrusion2" cut sketch "Sketch3" against normal through all contours L6 L7 L5 | L0 L8 L6 | L1 L7 L8 | L7 L8 L4 | L7 L2 L6 | L6 L3 L8
equation "\"d0\" = da_da"
equation "\"d3\" = da_d"
equation "\"d15\" = da_aw"
equation "\"d19\" = da_aw"
equation "\"da_da\" = 75.438"
equation "\"da_d\" = 73.025"
equation "\"da_aw\" = 28.575"
body "Solid1"
body "Srf1"
